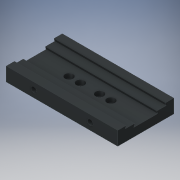
# Autodesk Inventor part: czescuchwytu
Saved by Autodesk Inventor 2019 (Build 230136000, 136)
## iProperties
Created: 2020-08-30
Part Number: czescuchwytu
Material: Iron, Cast
Document SubType Name: Modeling
Designer: estee
Density: 7.15 g/cm^3
Appearance: Iron Gray
Author: estee
Autodesk Inventor part; units mm, degrees
ref_plane "YZ Plane" through (0, 0, 0) normal (1, 0, 0) x (0, 1, 0)
ref_plane "XZ Plane" through (0, 0, 0) normal (0, 1, 0) x (-1, 0, 0)
ref_plane "XY Plane" through (0, 0, 0) normal (0, 0, 1) x (1, 0, 0)
sketch "Sketch1" plane through (0, 0, 0) normal (1, 0, 0) x (0, 1, 0)
  line L0 (-13.4609, 51.6064) -> (11.5391, 51.6064)
  line L1 (11.5391, -50.3936) -> (-13.4609, -50.3936)
  line L2 (-13.4609, -50.3936) -> (-13.4609, 51.6064)
  line L3 (-13.4609, 51.6064) -> (11.5391, -50.3936) construction
  line L4 (11.5391, 51.6064) -> (-13.4609, -50.3936) construction
  line L5 (1.5391, 22.1864) -> (1.5391, -20.9936)
  line L6 (7.1158, 37.8541) -> (11.5391, 36.6689)
  line L7 (6.5391, -36.6436) -> (11.5391, -35.3039)
  line L8 (6.5391, -36.6436) -> (13.9505, -36.6436) construction
  line L9 (1.5391, 22.1864) -> (7.1158, 20.6921)
  line L10 (1.5391, -20.9936) -> (6.5391, -19.6539)
  line L11 (7.1158, 37.8541) -> (7.1158, 20.6921)
  line L12 (6.5391, -19.6539) -> (6.5391, -36.6436)
  line L13 (11.5391, 51.6064) -> (11.5391, 36.6689)
  line L14 (11.5391, -35.3039) -> (11.5391, -50.3936)
  point P0 (-0.9609, 0.6064)
  dimension "d2" = 25
  dimension "d3" = 102
  dimension "d4" = 43.18
  dimension "d5" = 21.6
  dimension "d6" = 74.5
  dimension "d7" = 37.25
  dimension "d10" = 15
  dimension "d43" = 75
  constraints: 30 end point, 5 parallel, 3 vertical, 2 horizontal, 2 midpoint, 2 perpendicular
  measures "d2" distance of L1.start L1.end
  measures "d3" distance of L0.end L1.start
  measures "d4" distance of L5.start L5.end
  measures "d5" vertical distance of L5.end point (-0.961, 0.606)
  measures "d6" distance of L6.start L7.start
  measures "d7" vertical distance of point (-0.961, 0.606) L7.start
  measures "d10" angle of L8 L7
  measures "d43" angle of L11 L6
extrude "Extrusion1" add sketch "Sketch1" along normal blind 203
sketch "Sketch2" plane through (0, 1.5391, 22.1864) normal (0, 1, 0) x (1, 0, 0)
  line L0 (0, 72.58) -> (203, 72.58) projected
  point P0 (0, 22.1864)
  point P1 (63.3971, 21.58)
  point P2 (139.5971, 21.58)
  dimension "d14" = 76.2
  dimension "d15" = 63.4
  dimension "d44" = 51
  dimension "d45" = 51
  measures "d14" distance of point (139.597, 21.58) point (63.397, 21.58)
  measures "d15" distance of point (63.397, 21.58) point (0, 22.186)
  measures "d44" distance from line of L0 point (139.597, 21.58)
  measures "d45" distance from line of L0 point (63.397, 21.58)
hole "Hole1" at (63.3971, 1.5391, 0.6064) at (139.5971, 1.5391, 0.6064) direction (0, -1, 0) diameter 8.4 end through all counterbore diameter 15 counterbore depth 9
sketch "Sketch3" plane through (0, 1.5391, 22.1864) normal (0, 1, 0) x (1, 0, 0)
  line L0 (0, 72.58) -> (203, 72.58) projected
  line L1 (0, 0) -> (0, 43.18) projected
  point P0 (0, 22.1864)
  point P1 (84, 21.58)
  point P2 (119, 21.58)
  dimension "d23" = 35
  dimension "d46" = 51
  dimension "d47" = 51
  dimension "d48" = 84
  measures "d23" distance of point (84, 21.58) point (119, 21.58)
  measures "d46" distance from line of L0 point (84, 21.58)
  measures "d47" distance from line of L0 point (119, 21.58)
  measures "d48" distance from line of L1 point (84, 21.58)
hole "Hole2" at (84, 1.5391, 0.6064) at (119, 1.5391, 0.6064) direction (0, -1, 0) diameter 8.4 end through all counterbore diameter 15 counterbore depth 9
sketch "Sketch4" plane through (0, -13.4609, 51.6064) normal (0, 0, 1) x (1, 0, 0)
  line L0 (0, 0) -> (203, 0) projected
  line L1 (0, 0) -> (0, 25) projected
  line L2 (203, 25) -> (203, 0) projected
  point P0 (0, 13.4609)
  point P1 (50, 12.5)
  point P2 (153, 12.5)
  dimension "d32" = 12.5
  dimension "d33" = 12.5
  dimension "d34" = 50
  dimension "d35" = 50
  measures "d32" distance from line of L0 point (50, 12.5)
  measures "d33" distance from line of L0 point (153, 12.5)
  measures "d34" distance from line of L1 point (50, 12.5)
  measures "d35" distance from line of L2 point (153, 12.5)
hole "Hole3" at (50, -0.9609, 51.6064) at (153, -0.9609, 51.6064) direction (0, 0, -1) diameter 10 depth 10 tip angle 118
body "Solid1"
